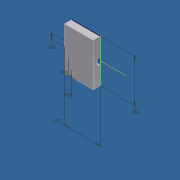
# Autodesk Inventor part: Wiring platform
Saved by Autodesk Inventor 2016 (Build 200138000, 138)
## iProperties
Created: 2014-06-19
Part Number: Wiring platform
Document SubType Name: Modeling
Designer: 121767
Density: 1 g/cm^3
Material: Generic
Appearance: Default
Author: 121767
Autodesk Inventor part; units mm, degrees
ref_plane "YZ Plane" through (0, 0, 0) normal (1, 0, 0) x (0, 1, 0)
ref_plane "XZ Plane" through (0, 0, 0) normal (0, 1, 0) x (-1, 0, 0)
ref_plane "XY Plane" through (0, 0, 0) normal (0, 0, 1) x (1, 0, 0)
sketch "Sketch1" plane through (0, 0, 0) normal (0, 0, 1) x (1, 0, 0)
  line L0 (-1.5141, -3) -> (-1.5141, 3)
  line L1 (-1.5141, 3) -> (-5.5141, 3)
  line L2 (-5.5141, 3) -> (-5.5141, -3)
  line L3 (-5.5141, -3) -> (-1.5141, -3)
  line L4 (-5.5141, -1.815) -> (-6.0141, -1.815)
  line L5 (-6.0141, -1.815) -> (-6.0141, -0.75)
  line L6 (-6.0141, -0.75) -> (-6.5141, -0.75)
  line L7 (-6.5141, -0.75) -> (-6.5141, 0)
  line L8 (-1.5141, 0) -> (-6.5141, 0)
  line L9 (-5.5141, 0) -> (-6.5141, 0)
  line L10 (-6.5141, 0) -> (-5.5141, 0)
  point P0 (0, 0)
  dimension "d0" = 0.5
  dimension "d1" = 1
  dimension "d2" = 5
  dimension "d18" = 0.75
  dimension "d19" = 6
  constraints: 24 end point, 5 parallel, 3 perpendicular, 3 point on line, 2 collinear, 2 midpoint, 1 vertical
  measures "d0" distance between parallel lines of L5 L7
  measures "d1" distance between parallel lines of L2 L7
  measures "d2" distance between parallel lines of L0 L7
  measures "d18" distance between parallel lines of L6 L8
  measures "d19" distance between parallel lines of L3 L1
extrude "Extrusion1" add sketch "Sketch1" along normal blind 1 contours L3 L2 L8 L0 | L8 L2 L1 L0
hole "Hole2" at (-5.5141, 0, 0) direction (1, 0, 0) diameter 1 depth 25.4 tip angle 118
body "Solid1"
